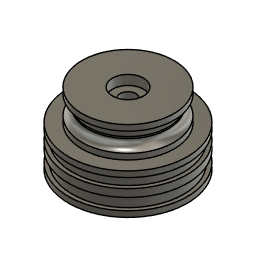
КолесоКроликВ3.1 (Autodesk Fusion 360 design; units mm, degrees)
Autodesk Fusion 360 part; units mm, degrees
sketch "Sketch1" plane through (0, 0, 0) normal (0, 1, 0) x (1, 0, 0)
  circle A0 centre (0, 0) radius 31
  circle A1 centre (0, 0) radius 8.1
  circle A2 centre (0, 0) radius 24
  circle A3 centre (0, 0) radius 4.1
  circle A4 centre (0, 0) radius 21
  line L0 (0, 0) -> (0, -24)
  line L1 (0, 0) -> (24, 0)
  line L2 (0, 0) -> (0, 24)
  line L3 (0, 0) -> (-24, 0)
  line L4 (0, 8) -> (-24, 8)
  line L5 (0, -8) -> (-24, -8)
  line L6 (-8, 0) -> (-8, -24)
  line L7 (8, 0) -> (8, -24)
  line L8 (0, -8) -> (22.6274, -8)
  line L9 (0, 8) -> (22.6274, 8)
  line L10 (8, 0) -> (8, 24)
  line L11 (-8, 0) -> (-8, 24)
  circle A5 centre (0, 0) radius 29
  dimension "d6" = 62
  dimension "d7" = 16.2
  dimension "d8" = 48
  dimension "d9" = 8.2
  dimension "d10" = 42
  dimension "d23" = 8
  dimension "d24" = -8
  dimension "d25" = 8
  dimension "d26" = -8
  dimension "d27" = 8
  dimension "d28" = -8
  dimension "d29" = 8
  dimension "d30" = -8
  dimension "d41" = 58
  constraint coincident A0.centre A1.centre
  constraint concentric A2 A3
  constraint concentric A1 A4
  constraint coincident A2 L0.end
  constraint vertical L0
  constraint coincident A2 L1.end
  constraint perpendicular L0 L1
  constraint coincident A2 L2.end
  constraint perpendicular L1 L2
  constraint coincident A2 L3.end
  constraint perpendicular L2 L3
  constraint concentric A4 A5
  constraint horizontal L5
  constraint coincident A2 L9.end
  constraint horizontal L9
  constraint coincident A2 L8.end
  constraint horizontal L8
  measures "d6" diameter of A0
  measures "d7" diameter of A1
  measures "d8" diameter of A2
  measures "d9" diameter of A3
  measures "d10" diameter of A4
  measures "d41" diameter of A5
extrude "Extrude1" add sketch "Sketch1" along normal blind 16 contours A1 A4 L1 L7 L8 | A1 A4 L1 L9 L10 | A1 L9 L10 | A1 L7 L8 | A1 A4 L2 L9 L10 | A4 L9 L10 | A1 A4 L0 L7 L8 | A4 L7 L8 | A1 A4 L2 L4 L11 | A1 A4 L0 L5 L6 | A1 L4 L11 | A1 L5 L6 | A1 A4 L3 L4 L11 | A4 L4 L11 | A1 A4 L3 L5 L6 | A4 L5 L6 makes body 1
extrude "Extrude2" add sketch "Sketch1" along normal blind 3 contours A2 A4 L1 L8 | A2 A4 L1 L9 | A2 A4 L9 L10 | A2 A4 L7 L8 | A2 A4 L2 L10 | A2 A4 L0 L7 | A2 A4 L2 L11 | A2 A4 L0 L6 | A2 A4 L4 L11 | A2 A4 L5 L6 | A2 A4 L3 L4 | A2 A4 L3 L5 bodies 1
extrude "Extrude3" add 1 faces at (22.8325, 3, 2.2356) along direction (0, 1, 0) blind 10 and the other way blind -13 on bodies 1 bodies 1
fillet "Fillet1" radius 5 2 edges at (-19.5789, 3, 7.5939) (-19.5789, 13, -7.5939) on bodies 1
extrude "Extrude4" add sketch "Sketch1" along normal blind 11 contours A1 L1 L10 | A1 L1 L7 | A1 A3 L1 L2 L9 L10 | A1 A3 L0 L1 L7 L8 | A1 L2 L9 | A1 L0 L8 | A1 L2 L4 | A1 A3 L2 L3 L4 L11 | A1 L0 L5 | A1 A3 L0 L3 L5 L6 | A1 L3 L11 | A1 L3 L6 bodies 1
extrude "Extrude5" add sketch "Sketch1" against normal blind 20 separate body contours A1 A4 L1 L7 L8 | A1 A4 L1 L9 L10 | A1 L9 L10 | A1 L7 L8 | A2 A4 L1 L8 | A2 A4 L1 L9 | A1 A4 L2 L9 L10 | A1 A4 L0 L7 L8 | A1 A4 L2 L4 L11 | A2 A4 L2 L10 | A1 A4 L0 L5 L6 | A2 A4 L0 L7 | A1 L4 L11 | A2 A4 L2 L11 | A1 L5 L6 | A2 A4 L0 L6 | A1 A4 L3 L4 L11 | A1 A4 L3 L5 L6 | A2 A4 L3 L4 | A2 A4 L3 L5 makes body 2
extrude "Extrude6" add sketch "Sketch1" against normal blind 15 contours A1 A3 L1 L2 L9 L10 | A1 A3 L0 L1 L7 L8 | A1 A3 L2 L3 L4 L11 | A1 A3 L0 L3 L5 L6 bodies 1 2
extrude "Extrude7" add sketch "Sketch1" against normal blind 20 separate body contours A0 | A4 L9 L10 | A4 L7 L8 | A2 A4 L9 L10 | A2 A4 L7 L8 | A4 L4 L11 | A2 A4 L4 L11 | A4 L5 L6 | A2 A4 L5 L6 | A5 makes body 3
extrude "Extrude8" add sketch "Sketch1" along normal blind -21 and the other way blind 20 contours A0 | A1 A4 L1 L7 L8 | A1 A4 L1 L9 L10 | A1 L9 L10 | A1 L7 L8 | A2 A4 L1 L8 | A2 A4 L1 L9 | A1 A4 L2 L9 L10 | A4 L9 L10 | A1 A4 L0 L7 L8 | A4 L7 L8 | A2 A4 L9 L10 | A2 A4 L7 L8 | A1 A4 L2 L4 L11 | A2 A4 L2 L10 | A1 A4 L0 L5 L6 | A2 A4 L0 L7 | A1 L4 L11 | A2 A4 L2 L11 | A1 L5 L6 | A2 A4 L0 L6 | A1 A4 L3 L4 L11 | A4 L4 L11 | A2 A4 L4 L11 | A1 A4 L3 L5 L6 | A4 L5 L6 | A2 A4 L5 L6 | A2 A4 L3 L4 | A2 A4 L3 L5 | A5 bodies 3
extrude "Extrude9" cut sketch "Sketch1" along normal blind -8 and the other way blind 3 contours A0 bodies 3
extrude "Extrude10" cut sketch "Sketch1" along normal blind -18 and the other way blind 12 contours A0 bodies 3
named bodies: "Колесо", "Шина"
